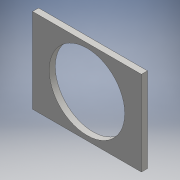
# Autodesk Inventor part: motor fixture
Saved by Autodesk Inventor 2016 (Build 200138000, 138)
## iProperties
Created: 2016-06-30
Part Number: motor fixture
Material: Generic
Document SubType Name: Modeling
Designer: hesaon
Density: 1 g/cm^3
Appearance: Default
Author: hesaon
Autodesk Inventor part; units mm, degrees
ref_plane "YZ Plane" through (0, 0, 0) normal (1, 0, 0) x (0, 1, 0)
ref_plane "XZ Plane" through (0, 0, 0) normal (0, 1, 0) x (-1, 0, 0)
ref_plane "XY Plane" through (0, 0, 0) normal (0, 0, 1) x (1, 0, 0)
sketch "Sketch1" plane through (0, 0, 0) normal (0, 1, 0) x (-1, 0, 0)
  line L0 (0, 0) -> (54, 0)
  line L1 (54, 0) -> (54, -42)
  line L2 (54, -42) -> (0, -42)
  line L3 (0, -42) -> (0, 0)
  circle A0 centre (27, -21) radius 18.75
  dimension "motorFixtureHeight" = 54
  dimension "motorFixtureWidth" = 42
  dimension "motorDiameter" = 37.5
  dimension "d3" = 27
  dimension "d4" = 21
  constraints: 8 end point, 2 parallel, 1 centre point, 1 horizontal, 1 perpendicular
  measures "motorFixtureHeight" distance of L1.end L2.end
  measures "motorFixtureWidth" distance of L0.end L1.end
  measures "motorDiameter" diameter of A0
  measures "d3" distance from line of L1 A0.centre
  measures "d4" distance from line of L0 A0.centre
extrude "Extrusion1" add sketch "Sketch1" along normal blind 3
equation "\"d3\" = 0.5 * motorFixtureHeight"
equation "\"d4\" = 0.5 * motorFixtureWidth"
body "Solid1"
